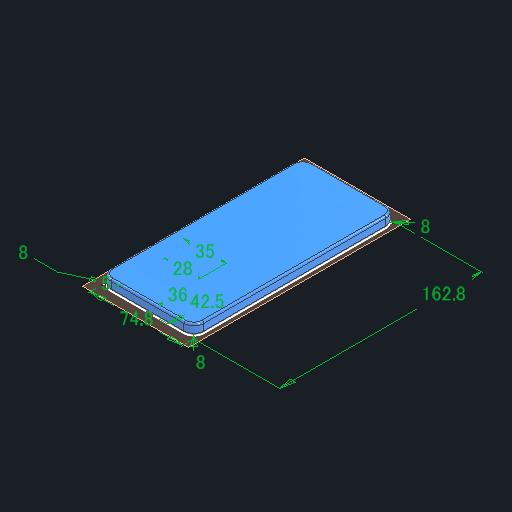
# Autodesk Inventor part: template
Saved by Autodesk Inventor 2025.2 (Build 292293000, 293)
## iProperties
Created: 2025-03-03
Part Number: template
Material: 一般
Document SubType Name: Sheet Metal
Designer: ktamu
Density: 1 g/cm^3
Sheet Metal Rule: Default_mm
Appearance: 既定
Author: ktamu
Autodesk Inventor part; units mm, degrees
ref_plane "YZ Plane" through (0, 0, 0) normal (1, 0, 0) x (0, 1, 0)
ref_plane "XY Plane" through (0, 0, 0) normal (0, 0, 1) x (1, 0, 0)
sketch "BASEsc" plane through (0, 0, 0) normal (0, 1, 0) x (-1, 0, 0)
  line L0 (-29.4, -81.4) -> (29.4, -81.4)
  line L1 (37.4, -73.4) -> (37.4, 73.4)
  line L2 (29.4, 81.4) -> (-29.4, 81.4)
  line L3 (-37.4, 73.4) -> (-37.4, -73.4)
  line L4 (-37.4, -81.4) -> (37.4, 81.4) construction
  line L5 (37.4, -81.4) -> (-37.4, 81.4) construction
  arc A0 (37.4, 73.4) -> (29.4, 81.4) centre (29.4, 73.4) ccw
  arc A1 (-29.4, 81.4) -> (-37.4, 73.4) centre (-29.4, 73.4) ccw
  arc A2 (-37.4, -73.4) -> (-29.4, -81.4) centre (-29.4, -73.4) ccw
  arc A3 (29.4, -81.4) -> (37.4, -73.4) centre (29.4, -73.4) ccw
  line L6 (25.4, 74.9) -> (7.4, 74.9)
  line L7 (2.4, 69.9) -> (2.4, 43.9)
  line L8 (7.4, 38.9) -> (25.4, 38.9)
  line L9 (30.4, 43.9) -> (30.4, 69.9)
  line L10 (30.4, 74.9) -> (2.4, 38.9) construction
  line L11 (2.4, 74.9) -> (30.4, 38.9) construction
  arc A4 (30.4, 69.9) -> (25.4, 74.9) centre (25.4, 69.9) ccw
  arc A5 (7.4, 74.9) -> (2.4, 69.9) centre (7.4, 69.9) ccw
  arc A6 (25.4, 38.9) -> (30.4, 43.9) centre (25.4, 43.9) ccw
  arc A7 (2.4, 43.9) -> (7.4, 38.9) centre (7.4, 43.9) ccw
  point P0 (0, 0)
  point P1 (16.4, 56.9)
  dimension "d0" = 74.8
  dimension "d1" = 162.8
  dimension "d2" = 8
  dimension "d3" = 8
  dimension "d4" = 8
  dimension "d7" = 28
  dimension "d8" = 36
  dimension "d9" = 5
  dimension "d26" = 42.5
  dimension "d27" = 35
  constraints: 24 end point, 16 point on circle, 16 point on line, 16 tangent, 8 centre point, 4 equal radius, 4 midpoint, 4 parallel, 2 horizontal, 2 perpendicular
  measures "d0" distance of L5.end L4.end
  measures "d1" distance of L5.end L4.start
  measures "d2" radius of A0
  measures "d3" radius of A1
  measures "d4" radius of A2
  measures "d7" distance of L11.end L10.end
  measures "d8" distance of L10.end L11.start
  measures "d9" radius of A4
  measures "d26" distance between parallel lines of L8 L2
  measures "d27" distance between parallel lines of L1 L7
extrude "押し出し1" add sketch "BASEsc" along normal blind 8.3 contours A2 L3 A1 L2 A0 L1 A3 L0 | A4 L9 A6 L8 A7 L7 A5 L6
extrude "押し出し2" add sketch "BASEsc" against normal blind 1 contours A4 L9 A6 L8 A7 L7 A5 L6
sketch "スケッチ2" plane through (-37.4, 0, -73.4) normal (-1, 0, 0) x (0, 0, 1)
  line L0 (143.2215, 4.15) -> (137.7549, 4.15) construction
  line L1 (0, 8.3) -> (146.8, 8.3) projected
  line L2 (132.2, 3.5) -> (113.4, 3.5)
  line L3 (112.8, 4.1) -> (112.8, 4.2)
  line L4 (113.4, 4.8) -> (132.2, 4.8)
  line L5 (132.8, 4.2) -> (132.8, 4.1)
  line L6 (132.8, 3.5) -> (112.8, 4.8) construction
  line L7 (112.8, 3.5) -> (132.8, 4.8) construction
  arc A0 (132.8, 4.2) -> (132.2, 4.8) centre (132.2, 4.2) ccw
  arc A1 (132.2, 3.5) -> (132.8, 4.1) centre (132.2, 4.1) ccw
  arc A2 (112.8, 4.1) -> (113.4, 3.5) centre (113.4, 4.1) ccw
  arc A3 (113.4, 4.8) -> (112.8, 4.2) centre (113.4, 4.2) ccw
  line L8 (154.8, 0) -> (154.8, 8.3) projected
  line L9 (105.3, 4.6243) -> (91.8, 4.6243)
  line L10 (91.8, 4.6243) -> (91.8, 3.6757)
  line L11 (91.8, 3.6757) -> (105.3, 3.6757)
  line L12 (105.3, 3.6757) -> (105.3, 4.6243)
  line L13 (105.3, 4.6243) -> (91.8, 3.6757) construction
  line L14 (91.8, 4.6243) -> (105.3, 3.6757) construction
  point P0 (73.4, 0)
  point P1 (140.4882, 4.15)
  point P2 (122.8, 4.15)
  point P3 (112.8, 4.15)
  point P4 (98.55, 4.15)
  point P5 (105.3, 4.15)
  dimension "d12" = 4.15
  dimension "d13" = 20
  dimension "d14" = 1.3
  dimension "d15" = 0.6
  dimension "d16" = 0.6
  dimension "d17" = 42
  dimension "d18" = 7.5
  dimension "d19" = 13.5
  constraints: 26 end point, 9 point on line, 8 point on circle, 8 tangent, 7 midpoint, 4 centre point, 4 parallel, 3 horizontal, 2 equal radius, 2 perpendicular
  measures "d12" distance from line of point (140.488, 4.15) L1
  measures "d13" distance of L6.end L7.end
  measures "d14" distance of L7.start L6.end
  measures "d15" radius of A0
  measures "d16" radius of A1
  measures "d17" distance from line of point (112.8, 4.15) L8
  measures "d18" distance of point (105.3, 4.15) point (112.8, 4.15)
  measures "d19" distance of L10.end L11.end
extrude "押し出し3" add sketch "スケッチ2" along normal blind 3
sketch "スケッチ3" plane through (29.4, 0, -81.4) normal (0, 0, -1) x (-1, 0, 0)
  line L0 (-8, 0) -> (-8, 8.3) projected
  line L1 (66.8, 0) -> (66.8, 8.3) projected
  line L2 (-8, 8.3) -> (66.8, 0) construction
  line L3 (66.8, 0) -> (66.8, 8.3)
  line L4 (0, 0) -> (-8, 0) projected
  line L5 (66.8, 8.3) -> (-8, 0) construction
  line L6 (24.4, 6.15) -> (34.4, 6.15)
  line L7 (34.4, 6.15) -> (34.4, 2.15)
  line L8 (34.4, 2.15) -> (24.4, 2.15)
  line L9 (24.4, 2.15) -> (24.4, 6.15)
  line L10 (24.4, 6.15) -> (34.4, 2.15) construction
  line L11 (34.4, 6.15) -> (24.4, 2.15) construction
  circle A0 centre (12.4, 4.15) radius 3.5
  point P0 (29.4, 0)
  point P1 (29.4, 4.15)
  point P2 (29.4, 4.15)
  dimension "d22" = 10
  dimension "d23" = 4
  dimension "d24" = 7
  dimension "d25" = 17
  constraints: 18 end point, 4 midpoint, 3 equal length, 1 centre point, 1 horizontal, 1 perpendicular
  measures "d22" distance of L7.end L8.end
  measures "d23" distance of L6.end L7.end
  measures "d24" diameter of A0
  measures "d25" distance of point (29.4, 4.15) A0.centre
extrude "押し出し4" cut sketch "スケッチ3" against normal blind 1
fillet "フィレット1" radius 1.5 8 edges at (35.0569, 8.3, -79.0569) (0, 8.3, -81.4) (-35.0569, 8.3, -79.0569) (-37.4, 8.3, 0) (-35.0569, 8.3, 79.0569) (0, 8.3, 81.4) (35.0569, 8.3, 79.0569) (37.4, 8.3, 0)
fillet "フィレット2" radius 1.5 8 edges at (-35.0569, 0, 79.0569) (0, 0, 81.4) (35.0569, 0, 79.0569) (37.4, 0, 0) (35.0569, 0, -79.0569) (0, 0, -81.4) (-35.0569, 0, -79.0569) (-37.4, 0, 0)
equation "\"BendRadius\" = Thickness"
equation "\"BendReliefWidth\" = Thickness"
equation "\"BendReliefDepth\" = 0.5 * Thickness"
equation "\"CornerReliefSize\" = 4 * Thickness"
equation "\"MinimumRemnant\" = 2 * Thickness"
equation "\"TransitionRadius\" = BendRadius"
equation "\"JacobiRadiusSize\" = BendRadius"
equation "\"GapSize\" = Thickness"
equation "\"Thickness\" = 0.5"
